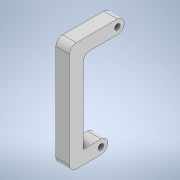
# Autodesk Inventor part: колено для сервы
Saved by Autodesk Inventor 2020.1 (Build 241239000, 239)
## iProperties
Created: 2022-04-03
Part Number: колено для сервы
Material: Типовые
Document SubType Name: Modeling
Designer: User
Density: 1 g/cm^3
Appearance: По умолчанию
Author: User
Autodesk Inventor part; units mm, degrees
ref_plane "YZ Plane" through (0, 0, 0) normal (1, 0, 0) x (0, 1, 0)
ref_plane "XZ Plane" through (0, 0, 0) normal (0, 1, 0) x (-1, 0, 0)
ref_plane "XY Plane" through (0, 0, 0) normal (0, 0, 1) x (1, 0, 0)
sketch "Эскиз1" plane through (0, 0, 0) normal (1, 0, 0) x (0, 1, 0)
  line L0 (0, 0) -> (10, 0)
  line L1 (10, 0) -> (10, 40)
  line L2 (10, 40) -> (0, 40)
  line L3 (0, 40) -> (0, 0)
  line L4 (10, 40) -> (-70, 40)
  line L5 (-70, 40) -> (-70, 30)
  line L6 (-70, 30) -> (10, 30)
  line L7 (10, 30) -> (10, 40)
  circle A0 centre (5, 5) radius 2
  line L8 (-70, 40) -> (-60, 40)
  line L9 (-60, 40) -> (-60, 12)
  line L10 (-60, 12) -> (-70, 12)
  line L11 (-70, 12) -> (-70, 40)
  circle A1 centre (-65, 17) radius 2
  point P0 (5, 0)
  point P1 (0, 40)
  point P2 (0, 30)
  point P3 (-70, 35)
  point P4 (-65, 12)
  point P5 (-60, 30)
  point P6 (-70, 30)
  dimension "d0" = 10
  dimension "d1" = 10
  dimension "d2" = 40
  dimension "d3" = 4
  dimension "d4" = 5
  dimension "d5" = 5
  dimension "d6" = 80
  dimension "d13" = 28
  dimension "d14" = 10
  dimension "d15" = 5
  constraints: 24 end point, 6 parallel, 3 horizontal, 3 midpoint, 3 perpendicular, 2 centre point
  measures "d0" distance of L0.start L0.end
  measures "d1" distance of L4.end L5.end
  measures "d2" distance of L2.end L0.start
  measures "d3" diameter of A0
  measures "d4" distance from line of L0 A0.centre
  measures "d5" distance from line of L1 A0.centre
  measures "d6" distance of L1.end L4.end
  measures "d13" distance of L10.end L4.end
  measures "d14" distance of L9.end L10.end
  measures "d15" distance from line of L10 A1.centre
extrude "Выдавливание1" add sketch "Эскиз1" along normal blind 10
fillet "Сопряжение1" radius 5 7 edges at (5, 0, 30) (5, 10, 40) (5, 10, 0) (5, 0, 0) (5, -70, 40) (5, -60, 12) (5, -70, 12)
